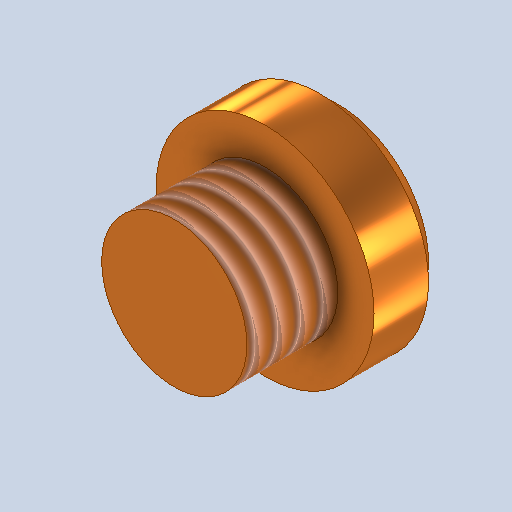
# Autodesk Inventor part: 153 part 2
Saved by Autodesk Inventor 2025.1 (Build 291241000, 241)
## iProperties
Created: 2024-08-01
Part Number: 153 part 2
Material: Gold
Document SubType Name: Modeling
Designer: ffogue
Density: 19.3 g/cm^3
Appearance: Metal 1600F Hot
Author: ffogue
Autodesk Inventor part; units mm, degrees
ref_plane "YZ Plane" through (0, 0, 0) normal (1, 0, 0) x (0, 1, 0)
ref_plane "XZ Plane" through (0, 0, 0) normal (0, 1, 0) x (-1, 0, 0)
ref_plane "XY Plane" through (0, 0, 0) normal (0, 0, 1) x (1, 0, 0)
sketch "Skizze1" plane through (0, 0, 0) normal (0, 0, 1) x (1, 0, 0)
  line L0 (0, 0) -> (0, 9)
  line L1 (0, 9) -> (6, 9)
  line L2 (6, 9) -> (6, 5)
  line L3 (6, 5) -> (4, 5)
  line L4 (4, 5) -> (4, 0)
  line L5 (4, 0) -> (0, 0)
  point P0 (5, 5)
  dimension "d0" = 8
  dimension "d1" = 12
  dimension "d2" = 5
  dimension "d3" = 4
  constraints: 12 end point, 5 perpendicular, 1 midpoint, 1 vertical
  measures "d0" diameter of L4 L0
  measures "d1" diameter of L2 L0
  measures "d2" distance between parallel lines of L5 L3
  measures "d3" distance from line of point (5, 5) L1
revolve "Umdrehung1" add sketch "Skizze1" angle 360 about axis through (0, 0, 0) along (0, 1, 0)
chamfer "Fasen1" distance 1 angle 45 1 edges at (-6, 9, 0)
thread "Gewinde1" size "M8x1.25" class "6g" standard "ISO Metric profile" full length
